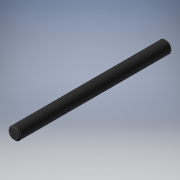
# Autodesk Inventor part: HHS25-PIN
Saved by Autodesk Inventor 2019 (Build 230136000, 136)
## iProperties
Created: 2024-01-05
Part Number: HHS25-PIN
Material: Generic
Catalog Web Link: www.cadenas.de
Description: HHS PIN-Butt Hinges
Vendor: MISUMI
Document SubType Name: Modeling
Designer: psAdmin
Manufacturer: MISUMI
Mass: 0.0783052 g
Surface Area: 1.61786 cm^2
Volume: 0.0783052 cm^3
Density: 1 g/cm^3
Appearance: PSOLRGB-175-175-175
Category: PARTsolutions
Company: MISUMI
Title: HHS25-PIN
Author: Cadenas PARTsolutions
Comments: Butt Hinges
PSOL_IDENT_0: {$CADENAS_DATA/23d-libs/misumi/metric/43_levers_knobs/parts_hhs/hhs_pin.prj},163 {VTYP=3D},{NB=HHS25
PSOL_IDENT_1: -PIN},{LINA=HHS25-PIN},{NN=HHS PIN},{DATE=04.06.2021 08:39:23},{GEOMDATE=17.02.2014 00:00:00},{VERSI
PSOL_IDENT_2: ON=},{LINEID=10},{WBVAR=LS},{WBNUMERIC=LS}  {NB=HHS25-PIN},{LINA=HHS25-PIN},{KT=DUMMY},{PN=HHS25},{N
PSOL_IDENT_3: O=25},{LS=25},{L111=25,30,40,50,65,75,90,100},{SN=A},{W=20},{W1=12},{W2=0},{L1=16},{C=2},{C1=3.8},{T
PSOL_IDENT_4: T=0.8},{DD=3.4},{NOD=3},{AL=9.8},{WT=6}
NB: HHS25-PIN
NN: HHS PIN
NT: Butt Hinges
NBSYN: $PN.-PIN
LINA: HHS25-PIN
CATALOG: Misumi
PN: HHS25
NO: 25
LS: 25
SN: A
W: 20
W1: 12
W2: 0
L1: 16
C: 2
C1: 3.8
TT: 0.8
DD: 3.4
NOD: 3
AL: 9.8
WT: 6
SUPPLIER: MISUMI
ARTICLENO: HHS25-PIN
BOMINFO: HHS25-PIN
CREATOR: CADENAS GmbH
Autodesk Inventor part; units mm, degrees
sketch "Sketch_1" plane through (0, 0, 0) normal (0, 1, 0) x (-1, 0, 0)
  line L0 (0, 0) -> (0, -25)
  line L1 (0, -25) -> (-0.8, -25)
  line L2 (-0.8, -25) -> (-1, -24.8)
  line L3 (-1, -24.8) -> (-1, -0.2)
  line L4 (-1, -0.2) -> (-0.8, 0)
  line L5 (-0.8, 0) -> (0, 0)
  line L6 (0, 0) -> (0, -25)
  constraints: 14 end point
revolve "Revolution1" add sketch "Sketch_1" angle 360 about axis through (0, 0, 0) along (0, 0, 1)
ref_plane "to_leaf_XY" through (0, 0, 0) normal (0, 0, 1) x (1, 0, 0)
ref_plane "to_leaf_YZ" through (0, 0, 0) normal (1, 0, 0) x (0, 1, 0)
ref_plane "to_leaf_ZX" through (0, 0, 0) normal (0, 1, 0) x (0, 0, 1)
body "Solid1"
